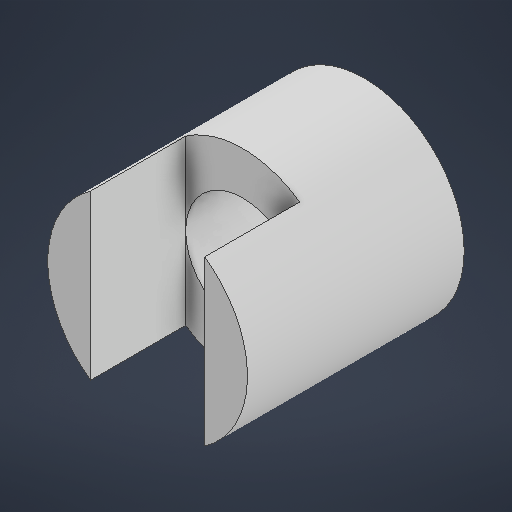
# Autodesk Inventor part: Part57
Saved by Autodesk Inventor 2027.1 (Build 311270010, 270A)
## iProperties
Created: 2026-10-02
Part Number: Part57
Material: Generic
Document SubType Name: Modeling
Designer: daniel
Density: 1 g/cm^3
Appearance: Default
Author: daniel
Autodesk Inventor part; units mm, degrees
ref_plane "YZ Plane" through (0, 0, 0) normal (1, 0, 0) x (0, 1, 0)
ref_plane "XZ Plane" through (0, 0, 0) normal (0, 1, 0) x (-1, 0, 0)
ref_plane "XY Plane" through (0, 0, 0) normal (0, 0, 1) x (1, 0, 0)
sketch "Sketch1" plane through (0, 0, 0) normal (0, 0, 1) x (1, 0, 0)
  circle A0 centre (0, 0) radius 3
  circle A1 centre (0, 0) radius 5.25
  line L0 (3, 4.3084) -> (3, -4.3084)
  line L1 (3, -3) -> (-3, -3)
  line L2 (-3, -4.3084) -> (-3, 4.3084)
  line L3 (-4.3084, 3) -> (4.3084, 3)
  dimension "d0" = 6
  dimension "d1" = 10.5
  constraints: 8 end point, 5 point on circle, 2 centre point, 2 coincident, 2 point on line, 1 parallel, 1 perpendicular
  measures "d0" diameter of A0
  measures "d1" diameter of A1
extrude "Extrusion1" add sketch "Sketch1" along normal blind 5 contours L0 L3 A1 | L0 A1 L3 | L2 A1 L3 | L3 A1 L2
extrude "Extrusion2" add sketch "Sketch1" against normal blind 6.4 contours L0 L1 A0 | L0 L3 A1 | A0 L3 L0 | A0 L2 L3 | L3 L2 A1 L0 | L1 L2 A0 | L1 L0 A1 L2 | L0 A1 L3 | L2 A1 L3 | L3 A1 L2
body "Solid1"
